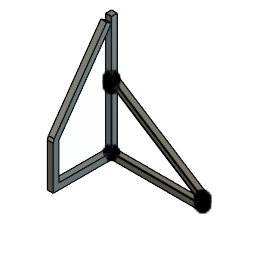
frame (Autodesk Fusion 360 design; units mm, degrees)
part number: 2026-02-08-14-37-26-257
Autodesk Fusion 360 part; units mm, degrees
sketch "Sketch1" plane through (0, 0, 0) normal (1, 0, 0) x (0, 0, -1)
  line L0 (-44.611, 20.8018) -> (-44.611, -99.8482)
  line L1 (-44.611, -99.8482) -> (126.839, -99.8482)
  line L2 (126.839, -99.8482) -> (126.839, 265.2768)
  line L3 (-44.611, 20.8018) -> (126.839, 265.2768)
  line L4 (-44.611, 20.8018) -> (-63.661, 20.8018)
  line L5 (-63.661, 20.8018) -> (-63.661, -101.6)
  line L6 (-63.661, -101.6) -> (-63.661, -120.65)
  line L7 (-63.661, -120.65) -> (127, -120.65)
  line L8 (127, -120.65) -> (146.05, -120.65)
  line L9 (146.05, -120.65) -> (146.05, 265.2768)
  line L10 (146.05, 265.2768) -> (146.05, 284.3268)
  line L11 (-44.611, 20.8018) -> (-60.2078, 31.7398)
  line L12 (126.839, 265.2768) -> (111.2422, 276.2148)
  line L13 (-60.2078, 31.7398) -> (111.2422, 276.2148)
  line L14 (-60.2078, 31.7398) -> (-63.661, 20.8018)
  line L15 (126.839, 265.2768) -> (126.839, 284.3268)
  line L16 (111.2422, 276.2148) -> (126.839, 284.3268)
  line L17 (126.839, 284.3268) -> (146.05, 284.3268)
  dimension "d1" = 120.65
  dimension "d2" = 171.45
  dimension "d3" = 365.125
  dimension "d4" = 19.05
  dimension "d5" = 19.05
  dimension "d6" = 19.05
  dimension "d7" = 180
  dimension "d8" = 19.05
  dimension "d9" = 19.05
  dimension "d10" = 19.05
  dimension "d11" = 19.05
  constraint vertical L0
  constraint perpendicular L0 L1
  constraint perpendicular L1 L2
  constraint perpendicular L0 L4
  constraint perpendicular L4 L5
  constraint perpendicular L4 L6
  constraint perpendicular L6 L7
  constraint perpendicular L6 L8
  constraint perpendicular L8 L9
  constraint perpendicular L3 L11
  constraint perpendicular L3 L12
  constraint parallel L2 L15
  constraint perpendicular L10 L17
  measures "d1" distance of L0.start L0.end
  measures "d2" distance of L0.end L1.end
  measures "d3" distance of L1.end L2.end
  measures "d4" distance of L0.start L4.end
  measures "d5" distance of L5.end L6.end
  measures "d6" distance of L7.end L8.end
  measures "d7" angle of L9 L10
  measures "d8" distance of L9.end L10.end
  measures "d9" distance of L0.start L11.end
  measures "d10" distance of L2.end L12.end
  measures "d11" distance of L2.end L15.end
extrude "Extrude1" add sketch "Sketch1" along normal blind 19.05 contours L3 L11 L12 L13 | L0 L1 L2 L4 L5 L6 L7 L8 L9 L10 L15 L17 | L4 L11 L14 makes body 1
sketch "Sketch2" plane through (19.05, 0, 0) normal (1, 0, 0) x (0, 0, -1)
  line L0 (-44.611, 20.8018) -> (126.839, 265.2768)
  line L1 (126.839, 265.2768) -> (111.2422, 276.2148)
  line L2 (111.2422, 276.2148) -> (-60.2078, 31.7398)
  line L3 (-60.2078, 31.7398) -> (-63.661, 20.8018)
  line L4 (-63.661, 20.8018) -> (-63.661, -120.65)
  line L5 (-63.661, -120.65) -> (146.05, -120.65)
  line L6 (146.05, -120.65) -> (146.05, 284.3268)
  line L7 (146.05, 284.3268) -> (126.839, 284.3268)
  line L8 (126.839, 284.3268) -> (126.839, 265.2768)
  line L9 (126.839, 265.2768) -> (126.839, -99.8482)
  line L10 (126.839, -99.8482) -> (-44.611, -99.8482)
  line L11 (-44.611, -99.8482) -> (-44.611, 20.8018)
  line L12 (126.839, -99.8482) -> (126.839, 90.6518)
  line L13 (126.839, 90.6518) -> (145.889, 90.6518)
  line L14 (145.889, 90.6518) -> (126.839, 90.6518)
  line L15 (126.839, 90.6518) -> (126.839, 109.7018)
  line L16 (126.839, 109.7018) -> (145.889, 109.7018)
  line L17 (145.889, 109.7018) -> (145.889, 90.6518)
  dimension "d14" = 190.5
  dimension "d15" = 19.05
  dimension "d16" = 19.05
  constraint coincident L9.end L10.start
  constraint perpendicular L10 L12
  constraint horizontal L13
  constraint horizontal L14
  constraint vertical L15
  constraint horizontal L16
  constraint vertical L17
  measures "d14" distance of L9.end L12.end
  measures "d15" distance of L12.end L13.end
  measures "d16" distance of L13.end L16.end
sketch "Sketch3" plane through (0, 0, 0) normal (0, 0, 1) x (1, 0, 0)
  line L0 (19.05, -99.8482, -126.839) -> (317.5, -99.8482, -126.839)
  line L1 (19.05, 90.6518, -126.839) -> (317.5, -99.8482, -126.839)
  line L2 (19.05, 109.7018, -126.839) -> (317.5085, -80.8037, -126.839)
  point P0 (19.05, -99.8482)
  point P1 (19.05, 90.6518)
  point P2 (19.05, 109.7018)
  dimension "d17" = 298.45
  dimension "d18" = 354.076
sketch "Sketch4" plane through (19.05, 0, 0) normal (1, 0, 0) x (0, 0, -1)
  line L0 (127, -101.6) -> (146.05, -101.6)
  line L1 (146.05, -101.6) -> (146.05, -120.65)
  line L2 (146.05, -120.65) -> (127, -120.65)
  line L3 (127, -120.65) -> (127, -101.6)
  dimension "d19" = 19.05
  dimension "d20" = 19.05
  constraint horizontal L0
  constraint vertical L1
  constraint horizontal L2
  constraint vertical L3
  measures "d19" distance of L0.start L0.end
  measures "d20" distance of L0.start L2.end
extrude "Extrude2" add sketch "Sketch4" along normal blind 298.45 separate body makes body 2
sketch "Sketch5" plane through (0, 0, 0) normal (0, 0, 1) x (1, 0, 0)
  line L0 (19.05, 109.7018, -126.839) -> (19.05, 90.6518, -126.839)
  line L1 (317.5085, -80.8037, -126.839) -> (317.5, -99.8482, -126.839)
  line L2 (19.05, 109.7018, -126.839) -> (19.05, 90.6518, -126.839)
  point P0 (19.05, 109.7018)
  point P1 (19.05, 90.6518)
  point P2 (317.5085, -80.8037)
  point P3 (317.5, -99.8482)
sketch "Sketch6" plane through (0, 0, 0) normal (0, 0, 1) x (1, 0, 0)
  line L0 (19.05, 90.6518, -145.889) -> (317.5, -101.6, -146.05)
  line L1 (19.05, 109.7018, -145.889) -> (317.5036, -82.5523, -146.05)
  line L2 (317.5036, -82.5523, -146.05) -> (317.5, -101.6, -146.05)
  line L3 (317.5085, -80.8037, -126.839) -> (317.5036, -82.5523, -146.05)
  line L4 (19.05, 109.7018, -145.889) -> (19.05, 90.6518, -145.889)
  point P0 (19.05, 90.6518)
  point P1 (317.5, -101.6)
  point P2 (19.05, 109.7018)
  point P3 (317.5085, -80.8037)
  dimension "d23" = 355.0115
  dimension "d24" = 355.0158
  measures "d23" distance of P0 P1
extrude "Extrude3" add sketch "Sketch6" along normal blind 19.05 separate body contours L0 L1 L2 L4 in plane through (-0.0787, 0, -145.8787) normal (0.000539, 0, 1) makes body 3
